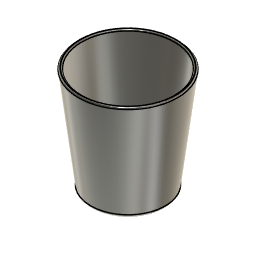
10409김태균_컵 (Autodesk Fusion 360 design; units mm, degrees)
Autodesk Fusion 360 part; units mm, degrees
sketch "스케치1" plane through (0, 0, 0) normal (0, 0, 1) x (1, 0, 0)
  circle A0 centre (0, 0) radius 35
  dimension "d1" = 70
  constraint coincident A0.centre origin
  measures "d1" diameter of A0
extrude "돌출1" add sketch "스케치1" along normal blind 100 draft 7
shell "쉘1" thickness 3 removed faces 1 at (-15.5835, -2.3488, 100)
fillet "필렛1" radius 1.4 2 edges at (-44.079, 17.0966, 100) (-41.261, 16.0036, 100)
fillet "필렛2" radius 4 2 edges at (-32.6315, -12.6565, 0) (-30.1569, -11.6967, 3)
